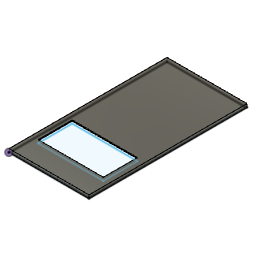
Case Parte de Cima (Autodesk Fusion 360 design; units mm, degrees)
Autodesk Fusion 360 part; units mm, degrees
sketch "Sketch1" plane through (0, 0, 0) normal (0, 0, 1) x (1, 0, 0)
  line L0 (0, 0) -> (38, 0)
  line L1 (38, 0) -> (38, 75)
  line L2 (38, 75) -> (0, 75)
  line L3 (0, 75) -> (0, 0)
  line L4 (34.1377, 10.6638) -> (3.2126, 10.6638)
  line L5 (3.2126, 10.6638) -> (3.2126, 26.8085)
  line L6 (3.2126, 26.8085) -> (34.1377, 26.8085)
  line L7 (34.1377, 26.8085) -> (34.1377, 10.6638)
  line L8 (0.5, 74.5) -> (0.5, 0.5)
  line L9 (0.5, 0.5) -> (37.5, 0.5)
  line L10 (37.5, 0.5) -> (37.5, 74.5)
  line L11 (37.5, 74.5) -> (0.5, 74.5)
  dimension "d1" = 38
  dimension "d2" = 75
  dimension "d9" = -0.5
  constraint horizontal L0
  constraint vertical L1
  constraint horizontal L2
  constraint vertical L3
  constraint coincident L0.start L3.end
  constraint horizontal L4
  constraint vertical L5
  constraint horizontal L6
  constraint vertical L7
  measures "d1" distance of L0.start L0.end
  measures "d2" distance of L0.start L2.end
extrude "Extrude1" add sketch "Sketch1" along normal blind 1.5 contours L0 L1 L2 L3 | L8 L9 L10 L11
extrude "Extrude3" cut sketch "Sketch1" along normal blind 1 contours L8 L9 L10 L11
